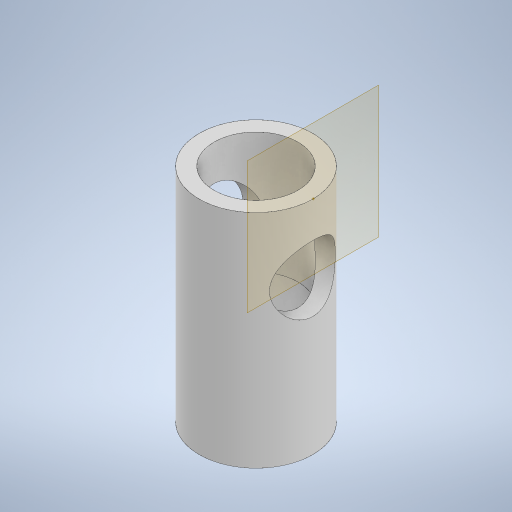
# Autodesk Inventor part: Mocowanie_do_wieszaka_w_kuchni
Saved by Autodesk Inventor 2024 (Build 280153000, 153)
## iProperties
Created: 2023-12-16
Part Number: Mocowanie_do_wieszaka_w_kuchni
Material: Generic
Document SubType Name: Modeling
Designer: Piter
Density: 1 g/cm^3
Appearance: Default
Author: Piter
Autodesk Inventor part; units mm, degrees
ref_plane "YZ Plane" through (0, 0, 0) normal (1, 0, 0) x (0, 1, 0)
ref_plane "XZ Plane" through (0, 0, 0) normal (0, 1, 0) x (-1, 0, 0)
sketch "Sketch1" plane through (0, 0, 0) normal (0, 1, 0) x (-1, 0, 0)
  circle A0 centre (0, 0) radius 9.5
  circle A1 centre (0, 0) radius 7
  circle A2 centre (0, 0) radius 3
  dimension "d0" = 19
  dimension "d1" = 14
  dimension "d6" = 6
  constraints: 3 centre point, 3 coincident
  measures "d0" diameter of A0
  measures "d1" diameter of A1
  measures "d6" diameter of A2
extrude "Extrusion1" add sketch "Sketch1" along normal blind 37 contours A0
extrude "Extrusion2" add sketch "Sketch1" along normal blind 3 contours A1
ref_plane "Work Plane1" through (9.5, 37, 0) normal (1, 0, 0) x (0, 1, 0)
sketch "Sketch2" plane through (9.5, 37, 0) normal (1, 0, 0) x (0, 1, 0)
  circle A0 centre (-11.5, 0) radius 5.5
  line L0 (0, -9.5) -> (0, 9.5) projected
  point P0 (-37, 0)
  point P1 (-6, 0)
  point P2 (0, 0)
  dimension "d7" = 11
  dimension "d9" = 6
  constraints: 1 horizontal alignment, 1 midpoint, 2 other
  measures "d9" distance of point (-6, 0) point (0, 0)
extrude "Extrusion3" cut sketch "Sketch2" against normal through all
chamfer "Chamfer2" distance 13.75 distance2 2.5 1 edges at (7, 3, 0) measured on face at (3.14, 21.6954, -6.2562)
body "Solid1"
